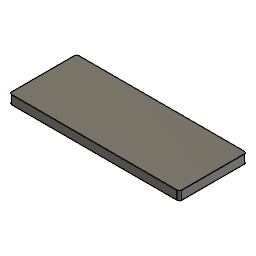
Keyboard Case (Autodesk Fusion 360 design; units mm, degrees)
part number: 2026-03-20-22-55-26-923
Autodesk Fusion 360 part; units mm, degrees
sketch "Szkic1" plane through (0, 0, 0) normal (0, 0, 1) x (1, 0, 0)
sketch "Szkic2" plane through (0, 0, 0) normal (0, 1, 0) x (1, 0, 0)
  line L0 (-150, 0) -> (-119, 0)
  line L1 (0, 0) -> (-310, 0)
  line L2 (-310, 0) -> (-310, -118)
  line L3 (-310, -118) -> (0, -118)
  line L4 (0, -118) -> (0, 0)
  line L5 (4, -117.5) -> (4, -0.5)
  line L6 (-0.5, 4) -> (-309.5, 4)
  line L7 (-314, -0.5) -> (-314, -117.5)
  line L8 (-309.5, -122) -> (-0.5, -122)
  arc A0 (4, -0.5) -> (-0.5, 4) centre (-0.5, -0.5) ccw
  arc A1 (-0.5, -122) -> (4, -117.5) centre (-0.5, -117.5) ccw
  arc A2 (-314, -117.5) -> (-309.5, -122) centre (-309.5, -117.5) ccw
  arc A3 (-309.5, 4) -> (-314, -0.5) centre (-309.5, -0.5) ccw
  dimension "d1" = 31
  dimension "d2" = 118
  dimension "d3" = 4.5
  constraint horizontal L0
  constraint coincident L1.start L4.end
  constraint parallel L0 L1
  constraint perpendicular L1 L2
  constraint perpendicular L2 L3
  constraint perpendicular L1 L4
  constraint parallel L4 L5
  constraint perpendicular L5 L6
  constraint perpendicular L3 L7
  constraint perpendicular L5 L8
  constraint tangent L5 A0
  constraint tangent L6 A0
  constraint tangent L5 A1
  constraint tangent L8 A1
  constraint equal A0 A1
  constraint tangent L7 A2
  constraint tangent L8 A2
  constraint equal A0 A2
  constraint tangent L6 A3
  constraint tangent L7 A3
  constraint equal A0 A3
  measures "d1" distance of L0.start L0.end
  measures "d2" distance of L1.end L2.end
  measures "d3" radius of A0
sketch "Szkic3" plane through (0, 0, 0) normal (0, 1, 0) x (1, 0, 0)
sketch "Szkic4" plane through (0, 0, 0) normal (0, 1, 0) x (1, 0, 0)
  line L0 (-0.5, 4) -> (-309.5, 4)
  line L1 (0, 0) -> (-310, 0)
  line L2 (-25, 4) -> (-25, 0)
  line L3 (-50, 4) -> (-50, 0)
  constraint coincident L0 L2.start
  constraint coincident L1 L2.end
  constraint perpendicular L1 L2
  constraint coincident L0 L3.start
  constraint coincident L1 L3.end
  constraint perpendicular L1 L3
extrude "Wyciągnięcie proste1" add sketch "Szkic2" against normal blind 12.5
sketch "Szkic5" plane through (0, 0, 0) normal (0, 1, 0) x (1, 0, 0)
  line L0 (0, 0) -> (-310, 0)
  line L1 (-310, 0) -> (-310, -120)
  line L2 (-310, -120) -> (0, -120)
  line L3 (0, -120) -> (0, 0)
  constraint coincident L0.start L3.end
  constraint horizontal L0
  constraint perpendicular L0 L1
  constraint perpendicular L1 L2
  constraint perpendicular L2 L3
sketch "Szkic6" plane through (0, 0, 0) normal (0, 1, 0) x (1, 0, 0)
extrude "Wyciągnięcie proste2" add sketch "Szkic5" against normal blind 3
extrude "Wyciągnięcie proste3" cut sketch "Szkic4" against normal blind 13
move_face "Odsuń powierzchnie1" offset 4 2 faces at (-120, 0, 81.3333) (-33.3333, -1, 0)
